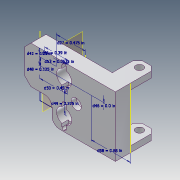
# Autodesk Inventor part: J005823
Saved by Autodesk Inventor 2015 SP1 (Build 190203100, 203)
## iProperties
Created: 2016-08-29
Material: ALUMINUM, 6061-T651
Vendor: HHMI: JRC - ID&F
Document SubType Name: Modeling
Designer: ARNOLDJ
Density: 2.7 g/cm^3
Appearance: Metal-AL-6061 (Machined)
Part Number: J005823
Description: ANGLE ADJ LOWER
Project: P-260102
RuleStatus: InUse
AfterDocSave0: file://Part Number Cleaner
LAB/DEPT: HANTMAN (LAB)
REQUESTING SCIENTIST: HANTMAN, ADAM
SURFACE ROUGHNESS: 63 Ra
DESIGN DEPARTMENT: HHMI: JRC - ID&F
SPECIAL FINISH: NONE
ALTERED ITEM PART NUMBER: N/A
ALTERED ITEM VENDOR: N/A
ALTERED ITEM DESCRIPTION: N/A
Revision Number: -
Autodesk Inventor part; units mm, degrees
ref_plane "XZ Plane" through (0, 0, 0) normal (0, 1, 0) x (-1, 0, 0)
ref_plane "XY Plane" through (0, 0, 0) normal (0, 0, 1) x (1, 0, 0)
sketch "Sketch1" plane through (0, 0, 0) normal (0, 0, 1) x (1, 0, 0)
  line L0 (0, 17.78) -> (0, -17.78) projected
  line L1 (-26.67, 0) -> (26.67, 0) projected
  line L2 (19.05, -12.7) -> (-19.05, -12.7)
  line L3 (-19.05, -12.7) -> (-19.05, 12.7)
  line L4 (-19.05, 12.7) -> (19.05, 12.7)
  line L5 (19.05, 12.7) -> (19.05, -12.7)
  line L6 (19.05, -12.7) -> (-19.05, 12.7) construction
  line L7 (-19.05, -12.7) -> (19.05, 12.7) construction
  point P0 (0, 0)
  dimension "d0" = 25.4
  dimension "d1" = 38.1
  constraints: 12 end point, 2 midpoint, 2 parallel, 1 horizontal, 1 perpendicular
  measures "d0" distance of L2.end L3.end
  measures "d1" distance of L3.end L4.end
extrude "Extrusion1" add sketch "Sketch1" along normal blind 6.35
sketch "Sketch2" plane through (0, 0, 0) normal (0, 0, 1) x (1, 0, 0)
  line L0 (0, 13.335) -> (0, -13.335) projected
  line L1 (19.05, -12.7) -> (19.05, 12.7) projected
  line L2 (-19.05, -12.7) -> (19.05, -12.7) projected
  point P0 (0, 0)
  point P1 (2.54, 0)
  point P2 (-12.065, 3.175)
  dimension "d27" = 12.065
  dimension "d46" = 0
  dimension "d48" = 3.175
  dimension "d58" = 16.51
  measures "d27" distance from line of L0 point (-12.065, 3.175)
  measures "d46" vertical distance of point (0, 0) point (2.54, 0)
  measures "d48" vertical distance of point (-12.065, 3.175) point (0, 0)
  measures "d58" distance from line of point (2.54, 0) L1
hole "Hole1" at (2.54, 0, 0) direction (0, 0, 1) diameter 4.318 end through all counterbore diameter 7.9502 counterbore depth 4.1656 clearance for "Socket Head Cap Screw" size "#8" standard "Ansi Unified Screw Threads"
sketch "Sketch3" plane through (0, 0, 0) normal (0, 0, 1) x (1, 0, 0)
  line L0 (19.05, -12.7) -> (19.05, 12.7) projected
  line L1 (19.05, 12.7) -> (-19.05, 12.7) projected
  line L2 (-19.05, -12.7) -> (19.05, -12.7) projected
  line L3 (0, 13.335) -> (0, -13.335) projected
  line L4 (-26.67, 0) -> (26.67, 0) projected
  line L5 (19.05, 12.7) -> (11.43, 12.7)
  line L6 (11.43, 12.7) -> (11.43, 10.16)
  line L7 (11.43, 10.16) -> (19.05, 10.16)
  line L8 (19.05, 10.16) -> (19.05, 12.7)
  line L9 (19.05, -12.7) -> (11.43, -12.7)
  line L10 (11.43, -12.7) -> (11.43, -10.16)
  line L11 (11.43, -10.16) -> (19.05, -10.16)
  line L12 (19.05, -10.16) -> (19.05, -12.7)
  point P0 (0, 0)
  dimension "d12" = 2.54
  dimension "d13" = 2.54
  dimension "d14" = 20.32
  dimension "d26" = 7.62
  constraints: 16 end point, 4 parallel, 2 horizontal, 2 perpendicular, 1 point on line
  measures "d12" distance of L9.end L10.end
  measures "d13" distance of L5.end L6.end
  measures "d14" distance between parallel lines of L11 L7
  measures "d26" distance of L6.end L7.end
extrude "Extrusion2" add sketch "Sketch3" against normal blind 10.668 contours L2 L10 L11 L0 | L7 L6 L1 L0
sketch "Sketch4" plane through (-19.05, 12.7, 6.35) normal (0, 1, 0) x (1, 0, 0)
  line L0 (19.05, 20.4216) -> (19.05, -3.4036) projected
  line L1 (45.72, 6.35) -> (-7.62, 6.35) projected
  line L2 (30.48, 17.018) -> (38.1, 17.018) projected
  line L3 (30.48, 6.35) -> (30.48, 17.018) projected
  line L4 (38.1, 0) -> (38.1, 17.018) projected
  line L5 (38.1, 0) -> (0, 0) projected
  point P0 (19.05, 6.35)
  point P1 (34.29, 13.97)
  dimension "d17" = 3.81
  dimension "d18" = 3.81
  dimension "d36" = 13.97
  dimension "d62" = 3.048
  measures "d17" distance from line of point (34.29, 13.97) L3
  measures "d18" distance from line of L4 point (34.29, 13.97)
  measures "d36" distance from line of point (34.29, 13.97) L5
  measures "d62" distance from line of point (34.29, 13.97) L2
hole "Hole2" at (15.24, 12.7, -7.62) direction (0, -1, 0) diameter 3.1877 end through all
hole "Hole3" [suppressed]
chamfer "Chamfer1" distance 1.905 angle 45 4 edges at (11.43, -11.43, -10.668) (19.05, -11.43, -10.668) (19.05, 11.43, -10.668) (11.43, 11.43, -10.668)
fillet "Fillet1" [suppressed]
sketch "Sketch5" plane through (0, 0, 0) normal (0, 0, -1) x (-1, 0, 0)
  line L0 (17.018, 0) -> (7.112, 0)
  line L1 (7.112, 0) -> (7.112, 6.35)
  line L2 (7.112, 6.35) -> (17.018, 6.35)
  line L3 (17.018, 6.35) -> (17.018, 0)
  line L4 (17.018, 0) -> (7.112, 6.35) construction
  line L5 (7.112, 0) -> (17.018, 6.35) construction
  line L6 (-11.43, -12.7) -> (19.05, -12.7) projected
  line L7 (19.05, -12.7) -> (19.05, 12.7) projected
  line L8 (19.05, -12.7) -> (7.62, -12.7)
  line L9 (7.62, -12.7) -> (7.62, -3.175)
  line L10 (7.62, -3.175) -> (19.05, -3.175)
  line L11 (19.05, -3.175) -> (19.05, -12.7)
  circle A0 centre (7.9057, 6.35) radius 0.7937
  circle A1 centre (16.2242, 6.35) radius 0.7937
  circle A2 centre (7.9057, 0) radius 0.7937
  circle A3 centre (16.2242, 0) radius 0.7938
  point P0 (0, 0)
  point P1 (12.065, 3.175)
  dimension "d53" = 1.5875
  dimension "d41" = 9.906
  dimension "d42" = 6.35
  dimension "d49" = 9.525
  dimension "d50" = 11.43
  constraints: 20 end point, 4 horizontal alignment, 4 parallel, 4 point on line, 2 horizontal, 2 midpoint, 2 perpendicular, 8 other
  measures "d41" distance of L1.end L2.end
  measures "d42" distance of L2.end L0.start
  measures "d49" distance of L8.end L9.end
  measures "d50" distance of L9.end L10.end
extrude "Extrusion3" cut sketch "Sketch5" against normal blind 1.27 contours A2 L0 | A2 L1 A0 L2 A1 L3 A3 L0 | L0 A2 | A3 L0 | L0 A3 | A0 L2 | L2 A0 | A1 L2 | L2 A1
fillet "Fillet2" [suppressed]
extrude "Extrusion4" cut sketch "Sketch5" against normal up to next contours L9 L10 L7 L6
ref_plane "Work Plane2" through (-12.065, 3.175, 0) normal (1, 0, 0) x (0, 1, 0)
fillet "Fillet3" radius 3.175 1 edges at (-7.62, -3.175, 3.175)
chamfer "Chamfer2" distance 2.54 angle 45 1 edges at (-19.05, -3.175, 3.175)
chamfer "Chamfer3" distance 2.54 angle 45 1 edges at (-19.05, 12.7, 3.175)
fillet "Fillet4" radius 3.175 1 edges at (-7.62, -12.7, 3.175)
sketch "Sketch6" plane through (0, 0, 0) normal (0, 0, 1) x (1, 0, 0)
  line L0 (0, 17.78) -> (0, -17.78) projected
  point P0 (0, 0)
  point P1 (-2.54, 6.985)
  point P2 (-2.54, -6.985)
  dimension "d64" = 6.985
  dimension "d65" = 13.97
  dimension "d66" = 2.54
  constraints: 1 vertical alignment
  measures "d64" vertical distance of point (0, 0) point (-2.54, 6.985)
  measures "d65" distance of point (-2.54, 6.985) point (-2.54, -6.985)
  measures "d66" distance from line of point (-2.54, 6.985) L0
hole "Hole4" at (-2.54, -6.985, 0) at (-2.54, 6.985, 0) direction (0, 0, 1) diameter 6.35 end through all
sketch "Sketch7" plane through (0, 0, 6.35) normal (0, 0, 1) x (1, 0, 0)
  circle A0 centre (-2.54, 6.985) radius 3.175 projected
  circle A1 centre (-2.54, -6.985) radius 3.175 projected
  line L0 (-1.651, 1.778) -> (-3.429, 1.778)
  line L1 (-3.429, 1.778) -> (-3.429, 12.192)
  line L2 (-3.429, 12.192) -> (-1.651, 12.192)
  line L3 (-1.651, 12.192) -> (-1.651, 1.778)
  line L4 (-1.651, 1.778) -> (-3.429, 12.192) construction
  line L5 (-3.429, 1.778) -> (-1.651, 12.192) construction
  line L6 (-3.429, -12.192) -> (-1.651, -12.192)
  line L7 (-1.651, -12.192) -> (-1.651, -1.778)
  line L8 (-1.651, -1.778) -> (-3.429, -1.778)
  line L9 (-3.429, -1.778) -> (-3.429, -12.192)
  line L10 (-3.429, -12.192) -> (-1.651, -1.778) construction
  line L11 (-1.651, -12.192) -> (-3.429, -1.778) construction
  circle A2 centre (2.54, 0) radius 2.159 projected
  point P0 (0, 0)
  dimension "d74" = 1.778
  dimension "d75" = 10.414
  dimension "d76" = 1.778
  dimension "d77" = 10.414
  constraints: 24 end point, 4 midpoint, 4 parallel, 2 horizontal, 2 perpendicular
  measures "d74" distance of L1.end L2.end
  measures "d75" distance of L0.end L1.end
  measures "d76" distance of L7.end L8.end
  measures "d77" distance between parallel lines of L8 L6
extrude "Extrusion5" cut sketch "Sketch7" against normal blind 2.54 contours L3 A0 L1 | A0 L1 L2 L3 | L3 L0 L1 A0 | L7 A1 L9 | A1 L9 L8 L7 | L7 L6 L9 A1
fillet "Fillet5" radius 0.7937 8 edges at (-3.429, 12.192, 5.08) (-1.651, 12.192, 5.08) (-3.429, 1.778, 5.08) (-1.651, 1.778, 5.08) (-3.429, -1.778, 5.08) (-1.651, -1.778, 5.08) (-3.429, -12.192, 5.08) (-1.651, -12.192, 5.08)
chamfer "Chamfer4" distance 0.889 angle 45 2 edges at (-2.54, -10.16, 0) (-2.54, 3.81, 0)
body "Solid1"
